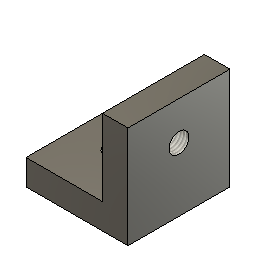
Profil Tutucu L (Autodesk Fusion 360 design; units mm, degrees)
Autodesk Fusion 360 part; units mm, degrees
sketch "Eskiz1" plane through (0, 0, 0) normal (0, 1, 0) x (1, 0, 0)
  circle A0 centre (15, -20) radius 4.5
  line L0 (0, 0) -> (30, 0)
  line L1 (30, 0) -> (30, -40)
  line L2 (30, -40) -> (0, -40)
  line L3 (0, -40) -> (0, 0)
  line L4 (30, 0) -> (40, 0)
  line L5 (40, 0) -> (40, -40)
  line L6 (40, -40) -> (30, -40)
  line L7 (30, -40) -> (30, 0)
  dimension "d3" = 9
  dimension "d13" = 40
  dimension "d25" = 10
  dimension "d31" = 30
  constraint horizontal L0
  constraint vertical L1
  constraint horizontal L2
  constraint vertical L3
  constraint coincident L0.start L3.end
  constraint horizontal L4
  constraint vertical L5
  constraint horizontal L6
  constraint vertical L7
  measures "d3" diameter of A0
  measures "d13" distance of L0.start L2.end
  measures "d25" distance of L0.end L4.end
  measures "d31" distance of L0.start L0.end
extrude "Ekstrüde Et9" add sketch "Eskiz1" along normal blind 10 contours A0 | L0 L1 L2 L3 L7
extrude "Ekstrüde Et10" add sketch "Eskiz1" along normal blind 40 contours L1 L4 L5 L6 L7
sketch "Eskiz4" plane through (30, 0, 0) normal (-1, 0, 0) x (0, 0, 1)
  line L0 (0, 10) -> (40, 10)
  line L1 (40, 10) -> (40, 40)
  line L2 (40, 40) -> (0, 40)
  line L3 (0, 40) -> (0, 10)
  circle A0 centre (20, 25) radius 4.5
  dimension "d36" = 9
  dimension "d37" = 15
  measures "d36" diameter of A0
  measures "d37" distance of L2 A0.centre
hole "Delik1" at (15.0452, 0, 20.1858) direction (0, 1, 0) diameter 7.779 depth 18 tip angle 118
thread "Diş3" "ISO Metric profile 9.0 M9x1.25 6H" thread offset 0 thread depth 10
hole "Delik2" at (30, 25, 20) direction (1, 0, 0) diameter 7.779 depth 18 tip angle 118
thread "Diş4" "ISO Metric profile 9.0 M9x1.25 6H" thread offset 0 thread depth 10
